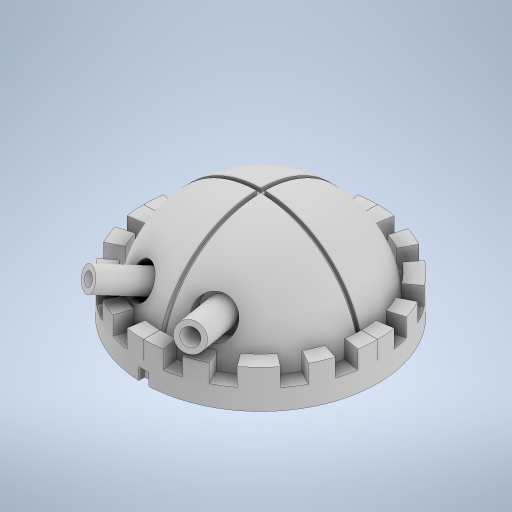
# Autodesk Inventor part: 屋頂-1
Saved by Autodesk Inventor 2024 (Build 280153000, 153)
## iProperties
Created: 2024-05-18
Part Number: 屋頂-1
Material: 一般
Document SubType Name: Modeling
Designer: User
Density: 1 g/cm^3
Appearance: 預設
Author: User
Autodesk Inventor part; units mm, degrees
sketch "草圖1" plane through (0, 0, 0) normal (0, 1, 0) x (-1, 0, 0)
  circle A0 centre (0, 0) radius 25
  circle A1 centre (0, 0) radius 29
  line L0 (25, 0) -> (-25, 0)
  dimension "d0" = 50
  dimension "d1" = 58
  constraints: 2 centre point, 2 coincident, 2 end point, 2 point on circle
  measures "d0" diameter of A0
  measures "d1" diameter of A1
revolve "迴轉1" add sketch "草圖1" angle 180 about axis through (-25, 0, 0) along (1, 0, 0) picked at (-2.955, -7.7918) contours A0 L0
sketch "草圖2" plane through (0, 0, 0) normal (0, -1, 0) x (1, 0, 0)
  circle A0 centre (0, 0) radius 25
  circle A1 centre (0, 0) radius 29
  dimension "d3" = 58
  constraints: 2 centre point, 2 coincident
  measures "d3" diameter of A1
extrude "擠出1" add sketch "草圖2" along normal blind 2 contours A0
extrude "擠出2" add sketch "草圖2" along normal blind 2 and the other way blind 3
sketch "草圖4" plane through (0, 0, 0) normal (1, 0, 0) x (0, 1, 0)
  arc A0 (0, -25) -> (0, 25) centre (0, 0) ccw projected
  line L0 (0, -25) -> (0, 25) projected
  line L1 (0, 25) -> (0, -25)
  arc A1 (0, -25) -> (0, 25) centre (0, 0) ccw
  arc A2 (0, -24) -> (0, 24) centre (0, 0) ccw
  point P0 (0, 24)
  dimension "d19" = 1
  constraints: 5 point on circle, 2 centre point, 2 concentric, 2 end point, 2 point on line, 1 collinear
  measures "d19" radial gap between concentric circles of A0 A2
extrude "擠出4" cut sketch "草圖4" along normal mid plane 1 contours L0 A2 A0
sketch "草圖5" plane through (0, 0, 0) normal (0, 0, 1) x (1, 0, 0)
  arc A0 (25, 0) -> (0.5, 24.995) centre (0, 0) ccw projected
  line L0 (-0.5, 0) -> (-25, 0) projected
  arc A1 (25, 0) -> (-25, 0) centre (0, 0) ccw
  line L1 (25, 0) -> (0.5, 0) projected
  arc A2 (24, 0) -> (-24, 0) centre (0, 0) ccw
  dimension "d23" = 1
  constraints: 5 point on circle, 2 centre point, 2 point on line, 1 concentric
  measures "d23" radial gap between concentric circles of A1 A2
extrude "擠出5" cut sketch "草圖5" along normal mid plane 1
sketch "草圖7" plane through (0, 3, 0) normal (0, 1, 0) x (1, 0, 0)
  circle A0 centre (0, 0) radius 29
  line L0 (0, 0) -> (4.4889, -28.6505)
  line L1 (0, 0) -> (-4.5111, -28.647)
  line L2 (-0.0111, -36.2405) -> (-0.0111, 33.0256)
  line L3 (0, 0) -> (0.5, -0.5) projected
  circle A1 centre (0, 0) radius 29 projected
  line L4 (36.2405, -0.0111) -> (-33.0256, -0.0111)
  line L5 (0, 0) -> (28.6505, 4.4889)
  line L6 (0, 0) -> (28.647, -4.5111)
  line L7 (0.0111, 36.2405) -> (0.0111, -33.0256)
  line L8 (0, 0) -> (-4.4889, 28.6505)
  line L9 (0, 0) -> (4.5111, 28.647)
  line L10 (-36.2405, 0.0111) -> (33.0256, 0.0111)
  line L11 (0, 0) -> (-28.6505, -4.4889)
  line L12 (0, 0) -> (-28.647, 4.5111)
  line L13 (0, 0) -> (-9.0441, -27.5537)
  line L14 (0, 0) -> (-13.6914, -25.5646)
  line L15 (0, 0) -> (8.3956, -27.7581)
  line L16 (0, 0) -> (13.0882, -25.8785)
  line L17 (0, 0) -> (25.5646, -13.6914)
  line L18 (0, 0) -> (27.5537, -9.0441)
  line L19 (0, 0) -> (27.7581, 8.3956)
  line L20 (0, 0) -> (25.8785, 13.0882)
  line L21 (0, 0) -> (13.6914, 25.5646)
  line L22 (0, 0) -> (9.0441, 27.5537)
  line L23 (0, 0) -> (-8.3956, 27.7581)
  line L24 (0, 0) -> (-13.0882, 25.8785)
  line L25 (0, 0) -> (-25.5646, 13.6914)
  line L26 (0, 0) -> (-27.5537, 9.0441)
  line L27 (0, 0) -> (-27.7581, -8.3956)
  line L28 (0, 0) -> (-25.8785, -13.0882)
  line L29 (0, 0) -> (-17.9226, -22.7987)
  line L30 (0, 0) -> (-23.2126, -17.3831)
  line L31 (0, 0) -> (17.3831, -23.2126)
  line L32 (0, 0) -> (22.7987, -17.9226)
  line L33 (0, 0) -> (23.2126, 17.3831)
  line L34 (0, 0) -> (17.9226, 22.7987)
  line L35 (0, 0) -> (-17.3831, 23.2126)
  line L36 (0, 0) -> (-22.7987, 17.9226)
  arc A2 (-24.995, 0.5) -> (-25, 0) centre (0, 0) ccw projected
  circle A3 centre (0, 0) radius 25
  point P0 (-19.654, 15.4505)
  point P1 (-14.9855, 20.0109)
  point P2 (-11.2829, 22.3091)
  point P3 (-7.2376, 23.9294)
  point P4 (-23.7532, 7.7967)
  point P5 (-22.0384, 11.8029)
  point P6 (-24.6957, 3.8889)
  point P7 (-29, 0.0111)
  point P8 (-25, 0.0111)
  point P9 (-24.6987, -3.8697)
  point P10 (-25, -0.0111)
  point P11 (-29, -0.0111)
  point P12 (-22.3091, -11.2829)
  point P13 (-23.9294, -7.2376)
  point P14 (-15.4505, -19.654)
  point P15 (-20.0109, -14.9855)
  point P16 (-7.7967, -23.7532)
  point P17 (-11.8029, -22.0384)
  point P18 (3.8697, -24.6987)
  point P19 (0.0111, -25)
  point P20 (0.0111, -29)
  point P21 (-0.0111, -25)
  point P22 (-3.8889, -24.6957)
  point P23 (-0.0111, -29)
  point P24 (11.2829, -22.3091)
  point P25 (7.2376, -23.9294)
  point P26 (19.654, -15.4505)
  point P27 (14.9855, -20.0109)
  point P28 (23.7532, -7.7967)
  point P29 (22.0384, -11.8029)
  point P30 (25, -0.0111)
  point P31 (24.6957, -3.8889)
  point P32 (29, -0.0111)
  point P33 (24.6987, 3.8697)
  point P34 (25, 0.0111)
  point P35 (29, 0.0111)
  point P36 (22.3091, 11.2829)
  point P37 (23.9294, 7.2376)
  point P38 (15.4505, 19.654)
  point P39 (20.0109, 14.9855)
  point P40 (7.7967, 23.7532)
  point P41 (11.8029, 22.0384)
  point P42 (-3.8697, 24.6987)
  point P43 (-0.0111, 25)
  point P44 (-0.0111, 29)
  point P45 (0.0111, 25)
  point P46 (3.8889, 24.6957)
  point P47 (0.0111, 29)
  dimension "d27" = 58
  dimension "d26" = 9
  dimension "d28" = 4.5
  dimension "d31" = 360
  dimension "d33" = 10
  dimension "d36" = 360
  dimension "d38" = 15
  dimension "d39" = 10
  dimension "d40" = 10
  dimension "d43" = 360
  constraints: 72 end point, 4 coincident, 4 point on circle, 1 vertical, 100 other
  measures "d26" distance of L0.end L1.end
  measures "d28" distance from line of L2 L1.end
  measures "d33" angle of L13 L14
  measures "d38" angle of L29 L30
  measures "d39" angle of L14 L29
  measures "d40" angle of L28 L30
extrude "擠出6" add sketch "草圖7" along normal blind 4.5 contours A0 L10 A3 L5 | L19 A3 L20 A0 | L33 A3 L34 A0 | A0 L6 A3 L4 | A3 L8 A0 L2 | A3 L11 A0 L4 | L7 A0 L9 A3 | L10 A0 L12 A3 A2 | L13 A0 L14 A3 | L16 A0 L15 A3 | A3 L18 A0 L17 | A3 L22 A0 L21 | A3 L24 A0 L23 | A3 L26 A0 L25 | A3 L28 A0 L27 | L29 A0 L30 A3 | A3 L32 A0 L31 | A3 L36 A0 L35 | L0 A0 L7 A3 | A3 L2 A0 L1
ref_plane "工作平面3" through (0, 0, 29) normal (0, 0, 1) x (1, 0, 0)
sketch "草圖8" plane through (0, 0, 29) normal (0, 0, 1) x (1, 0, 0)
  line L0 (1.2503, 1) -> (-1.2497, 1)
  line L1 (-1.2497, 1) -> (-1.2497, -2)
  line L2 (-1.2497, -2) -> (1.2503, -2)
  line L3 (1.2503, -2) -> (1.2503, 1)
  line L4 (1.2503, 1) -> (-1.2497, -2) construction
  line L5 (-1.2497, 1) -> (1.2503, -2) construction
  line L6 (-29, -2) -> (29, -2) projected
  line L7 (0.0003, -0.3702) -> (0.0003, -0.658)
  point P0 (0.0003, -0.5)
  point P1 (0.0003, -2)
  dimension "d48" = 2.5
  dimension "d49" = 3
  constraints: 14 end point, 3 midpoint, 2 parallel, 2 point on line, 1 horizontal, 1 perpendicular, 1 vertical
  measures "d48" distance of L2.end L1.end
  measures "d49" distance of L1.end L0.end
extrude "擠出7" cut sketch "草圖8" against normal blind 1.5
ref_plane "工作平面4" through (0, 0, 0) normal (-0.3769, 0.2873, 0.8806) x (-0.6063, -0.7952, 0)
sketch "草圖9" plane through (0, 0, 0) normal (-0.3769, 0.2873, 0.8806) x (-0.6063, -0.7952, 0)
  circle A0 centre (-3.163, -2.8098) radius 1.5
  circle A1 centre (-3.163, -2.8098) radius 2.75
  point P0 (0, 0)
  dimension "d52" = 3
  dimension "d53" = 5.5
  constraints: 2 centre point, 1 coincident
  measures "d52" diameter of A0
  measures "d53" diameter of A1
extrude "擠出8" add sketch "草圖9" along normal blind 35
sketch "草圖10" plane through (-13.2412, 14.0726, 29.4878) normal (-0.3769, 0.2873, 0.8806) x (0.9193, 0, 0.3935)
  circle A0 centre (0, 0) radius 2.75
  circle A1 centre (0, 0) radius 4
  point P0 (0.5699, -4.1922)
  dimension "d56" = 5.5
  dimension "d57" = 8
  constraints: 2 centre point, 1 coincident
  measures "d56" diameter of A0
  measures "d57" diameter of A1
extrude "擠出9" cut sketch "草圖10" against normal blind 15
ref_plane "工作平面5" through (0, 0, 0) normal (-0.36, -0.2504, -0.8987) x (0.571, -0.8209, 0)
sketch "草圖11" plane through (0, 0, 0) normal (-0.36, -0.2504, -0.8987) x (0.571, -0.8209, 0)
  circle A0 centre (-4.9236, -3.5965) radius 2
  circle A1 centre (-4.9236, -3.5965) radius 3.25
  point P0 (0, 0)
  dimension "d60" = 4
  dimension "d61" = 6.5
  constraints: 2 centre point, 1 coincident
  measures "d60" diameter of A0
  measures "d61" diameter of A1
extrude "擠出10" add sketch "草圖11" against normal blind 35
sketch "草圖12" plane through (12.4415, 14.651, 29.8786) normal (0.36, 0.2504, 0.8987) x (0.9283, 0, -0.3718)
  circle A0 centre (0, 0) radius 4.5
  circle A1 centre (0, 0) radius 3.25
  point P0 (-0.4398, -6.0814)
  dimension "d64" = 9
  dimension "d65" = 6.5
  constraints: 2 centre point, 1 coincident
  measures "d64" diameter of A0
  measures "d65" diameter of A1
extrude "擠出11" cut sketch "草圖12" against normal blind 15
